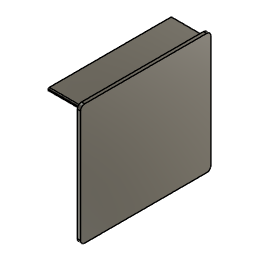
tapa+sensor (Autodesk Fusion 360 design; units mm, degrees)
Autodesk Fusion 360 part; units mm, degrees
sketch "Boceto1" plane through (0, 0, 0) normal (1, 0, 0) x (0, 1, 0)
  line L0 (-59, 101) -> (59, 101)
  line L1 (59, 101) -> (59, 0)
  line L2 (59, 0) -> (-59, 0)
  line L3 (-59, 0) -> (-59, 101)
  dimension "d4" = 101
  dimension "d5" = 118
  constraint horizontal L0
  constraint vertical L1
  constraint horizontal L2
  constraint vertical L3
  constraint midpoint origin L2
  measures "d4" distance of L0.start L2.end
  measures "d5" distance of L0.start L0.end
extrude "Extruir1" add sketch "Boceto1" along normal blind 29 makes body 1
sketch "Boceto2" plane through (0, 0, 0) normal (-1, 0, 0) x (0, -1, 0)
  line L0 (-59, 0) -> (59, 0)
  line L1 (59, 0) -> (59, 101)
  line L2 (59, 101) -> (-59, 101)
  line L3 (-59, 101) -> (-59, 0)
  line L4 (-62.5, -3.5) -> (-62.5, 111.2)
  line L5 (-62.5, 111.2) -> (-56, 111.2)
  line L6 (-56, 111.2) -> (-56, 108.2)
  line L7 (-56, 108.2) -> (-59.5, 108.2)
  line L8 (-59.5, 108.2) -> (-59.5, 104.5)
  line L9 (-59.5, 104.5) -> (-56, 104.5)
  line L10 (-56, 104.5) -> (-56, 101.5)
  line L11 (-56, 101.5) -> (-59.5, 101.5)
  line L12 (-59.5, 101.5) -> (-59.5, -0.5)
  line L13 (-59.5, -0.5) -> (0, -0.5)
  line L14 (-62.5, -3.5) -> (0, -3.5)
  line L15 (0, 2.5) -> (0, 20)
  line L16 (62.5, -3.5) -> (0, -3.5)
  line L17 (59.5, -0.5) -> (0, -0.5)
  line L18 (59.5, 101.5) -> (59.5, -0.5)
  line L19 (62.5, -3.5) -> (62.5, 111.2)
  line L20 (56, 101.5) -> (59.5, 101.5)
  line L21 (56, 104.5) -> (56, 101.5)
  line L22 (59.5, 104.5) -> (56, 104.5)
  line L23 (59.5, 108.2) -> (59.5, 104.5)
  line L24 (56, 108.2) -> (59.5, 108.2)
  line L25 (56, 111.2) -> (56, 108.2)
  line L26 (62.5, 111.2) -> (56, 111.2)
  line L27 (56, 111.2) -> (-56, 111.2)
  dimension "d10" = 0.5
  dimension "d11" = 3.7
  dimension "d12" = 3.5
  dimension "d13" = 0.5
  dimension "d14" = 0.5
  dimension "d15" = 3
  dimension "d16" = 3
  dimension "d17" = 3
  dimension "d18" = 3
  constraint vertical L8
  constraint perpendicular L8 L9
  constraint perpendicular L9 L10
  constraint vertical origin L13.end
  constraint vertical L13.end L14.end
  constraint horizontal L11
  constraint horizontal L7
  constraint horizontal L5
  constraint vertical L6
  constraint vertical L4
  constraint vertical L12
  constraint horizontal L14
  constraint horizontal L13
  constraint coincident L8 L11.end
  constraint coincident L6 L9.end
  constraint symmetric L4.start L15 L16.start
  constraint symmetric L4.end L15 L19.end
  constraint symmetric L5.end L15 L25.start
  constraint symmetric L6.end L15 L24.start
  constraint symmetric L7.end L15 L23.start
  constraint symmetric L8.end L15 L22.start
  constraint symmetric L9.end L15 L21.start
  constraint symmetric L10.end L15 L20.start
  constraint symmetric L11.end L15 L18.start
  constraint symmetric L12.end L15 L17.start
  constraint symmetric L13.end L15 L17.end
  constraint symmetric L14.end L15 L16.end
  measures "d10" distance of origin L13.end
  measures "d11" distance of L7.end L8.end
  measures "d12" distance of L6.end L7.end
  measures "d13" distance of L3 L12
  measures "d14" distance of L2 L11
  measures "d15" distance of L4 L12
  measures "d16" distance of L13 L14
  measures "d17" distance of L5.end L6.end
  measures "d18" distance of L9.end L10.end
extrude "Extruir2" add sketch "Boceto2" along normal blind 0 and the other way blind 31 separate body contours L4 L5 L6 L7 L8 L9 L10 L11 L12 L13 L14 L16 L17 L18 L19 L20 L21 L22 L23 L24 L25 L26 makes body 2
extrude "Extruir3" add sketch "Boceto2" along normal blind 3 contours L0 L1 L2 L3 | L4 L5 L6 L7 L8 L9 L10 L11 L12 L13 L14 L16 L17 L18 L19 L20 L21 L22 L23 L24 L25 L26 | L6 L7 L8 L9 L10 L11 L12 L13 L17 L18 L20 L21 L22 L23 L24 L25 L27 bodies 2
fillet "Empalme1" radius 4 4 edges at (14, 62.5, 111.2) (14, 62.5, -3.5) (14, -62.5, 111.2) (14, -62.5, -3.5) on bodies 2
fillet "Empalme2" radius 0.5 8 edges at (15.5, 56, 111.2) (15.5, 56, 101.5) (15.5, 56, 104.5) (15.5, 56, 108.2) (15.5, -56, 101.5) (15.5, -56, 108.2) (15.5, -56, 111.2) (15.5, -56, 104.5) on bodies 2
sketch "Boceto3" plane through (0, 0, 0) normal (0, 1, 0) x (1, 0, 0)
  line L0 (34.3, -111.2) -> (31.3, -111.2)
  line L1 (31.3, -111.2) -> (31.3, 3.5)
  line L2 (31.3, 3.5) -> (34.3, 3.5)
  line L3 (34.3, 3.5) -> (34.3, -111.2)
  line L4 (31.3, -107.85) -> (0.6, -107.85)
  line L5 (0.6, -107.85) -> (0.6, -104.85)
  line L6 (0.6, -104.85) -> (31.3, -104.85)
  line L7 (31.3, -104.85) -> (31.3, -107.85)
  line L8 (0, -108.2) -> (0, -104.5)
  line L9 (31, -108.2) -> (0, -108.2)
  point P0 (31, 3.5)
  point P1 (31, -111.2)
  dimension "d29" = 3
  dimension "d30" = 0.6
  dimension "d31" = 0.35
  dimension "d32" = 0.3
  dimension "d33" = 3
  constraint horizontal L0
  constraint vertical L1
  constraint horizontal L2
  constraint vertical L3
  constraint horizontal L4
  constraint vertical L5
  constraint horizontal L6
  constraint vertical L7
  constraint coincident L1 L4.start
  constraint coincident L2 P0
  constraint coincident L0 P1
  measures "d29" distance of L4.end L5.end
  measures "d30" distance of L5 L8
  measures "d31" distance of L4 L9
  measures "d32" distance of L1 P1
  measures "d33" distance of L0.start L0.end
extrude "Extruir4" add sketch "Boceto3" along normal mid plane 118 separate body contours L1 L4 L5 L6 L7 makes body 3
extrude "Extruir5" add sketch "Boceto3" along normal mid plane 124 contours L0 L1 L2 L3 L7 bodies 3
fillet "Empalme3" radius 4 4 edges at (32.8, 62, 111.2) (32.8, -62, 111.2) (32.8, -62, -3.5) (32.8, 62, -3.5) on bodies 3
fillet "Empalme4" radius 1.5 4 edges at (31.3, 0, 104.85) (31.3, -59, 106.35) (31.3, 0, 107.85) (31.3, 59, 106.35) on bodies 3
fillet "Empalme5" radius 1 8 edges at (15.2, 59, 107.85) (30.8607, 59.4393, 108.2893) (30.8607, 59.4393, 104.4107) (15.2, 59, 104.85) (30.8607, -59.4393, 108.2893) (15.2, -59, 107.85) (15.2, -59, 104.85) (30.8607, -59.4393, 104.4107) on bodies 3
hidden bodies 1 2
equation "largo = 29 mm"
equation "ancho = 118 mm"
equation "alto = 101 mm"
equation "d4 = alto"
equation "d5 = ancho"
equation "d6 = largo"
equation "d21 = largo + 2 mm"
equation "d36 = ancho"
equation "d38 = ancho + 6 mm"
